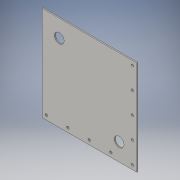
# Autodesk Inventor part: 1073-2017 Shooter Outside Plate Right
Saved by Autodesk Inventor 2016 (Build 200138000, 138)
## iProperties
Created: 2017-01-29
Part Number: 1073-2017 Shooter Outside Plate Right
Material: Generic
Document SubType Name: Modeling
Designer: rasmussenf
Density: 1 g/cm^3
Appearance: Default
Author: rasmussenf
Autodesk Inventor part; units mm, degrees
ref_plane "YZ Plane" through (0, 0, 0) normal (1, 0, 0) x (0, 1, 0)
ref_plane "XZ Plane" through (0, 0, 0) normal (0, 1, 0) x (-1, 0, 0)
ref_plane "XY Plane" through (0, 0, 0) normal (0, 0, 1) x (1, 0, 0)
sketch "Sketch1" plane through (0, 0, 0) normal (0, 0, 1) x (1, 0, 0)
  line L0 (0, 0) -> (279.4, 0)
  line L1 (279.4, 0) -> (279.4, 279.4)
  line L2 (279.4, 279.4) -> (0, 279.4)
  line L3 (0, 279.4) -> (0, 0)
  circle A0 centre (50.8, 228.6) radius 14.2875
  circle A1 centre (50.8, 228.6) radius 250.0376 construction
  circle A2 centre (227.6033, 51.7967) radius 14.2875
  line L4 (50.8, 228.6) -> (279.4, 0) construction
  dimension "d5" = 500.0752
  dimension "d0" = 279.4
  dimension "d1" = 279.4
  dimension "d2" = 28.575
  dimension "d3" = 228.6
  dimension "d4" = 228.6
  dimension "d6" = 28.575
  constraints: 10 end point, 2 centre point, 2 parallel, 1 coincident, 1 horizontal, 1 perpendicular, 1 point on line, 3 other
  measures "d0" distance of L1.end L2.end
  measures "d1" distance of L0.end L1.end
  measures "d2" diameter of A0
  measures "d3" distance from line of L1 A0.centre
  measures "d4" distance from line of A0.centre L0
  measures "d6" diameter of A2
extrude "Extrusion1" add sketch "Sketch1" along normal blind 3.175
sketch "Sketch2" plane through (0, 0, 3.175) normal (0, 0, 1) x (1, 0, 0)
  circle A0 centre (266.7, 12.7) radius 3.5687
  line L0 (0, 0) -> (279.4, 0) projected
  line L1 (279.4, 0) -> (279.4, 279.4) projected
  circle A1 centre (266.7, 76.2) radius 3.5687
  circle A2 centre (266.7, 139.7) radius 3.5687
  circle A3 centre (266.7, 203.2) radius 3.5687
  circle A4 centre (266.7, 266.7) radius 3.5687
  circle A5 centre (203.2, 12.7) radius 3.5687
  circle A6 centre (139.7, 12.7) radius 3.5687
  circle A7 centre (76.2, 12.7) radius 3.5687
  circle A8 centre (12.7, 12.7) radius 3.5687
  dimension "d9" = 7.1374
  dimension "d10" = 12.7
  dimension "d11" = 12.7
  dimension "d14" = 63.5
  dimension "d24" = 63.5
  constraints: 9 centre point, 1 horizontal, 1 vertical, 16 other
  measures "d9" diameter of A0
  measures "d10" distance from line of L0 A0.centre
  measures "d11" distance from line of L1 A0.centre
  measures "d14" distance of A0.centre A1.centre
  measures "d24" distance of A0.centre A5.centre
extrude "Extrusion2" cut sketch "Sketch2" against normal blind 3.175
body "Solid1"
